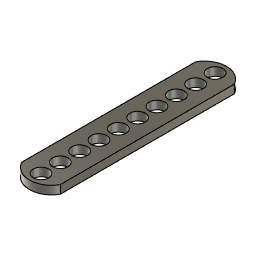
Cut_Link v2 (Autodesk Fusion 360 design; units mm, degrees)
Autodesk Fusion 360 part; units mm, degrees
sketch "Sketch1" plane through (0, 0, 0) normal (0, 0, 1) x (1, 0, 0)
  line L0 (0, 0) -> (0, 45) construction
  line L1 (0, 0) -> (-5, 0)
  line L2 (-5, 0) -> (-5, 45)
  line L3 (-5, 45) -> (0, 45)
  line L4 (5, 0) -> (5, 45)
  line L5 (0, 22.5) -> (9.3523, 22.5) construction
  arc A0 (5, 45) -> (-5, 45) centre (0, 42.289) ccw
  circle A1 centre (0, 45) radius 2
  arc A2 (-5, 0) -> (5, 0) centre (0, 2.711) ccw
  circle A3 centre (0, 0) radius 2
  circle A4 centre (0, 40) radius 2
  circle A5 centre (0, 35) radius 2
  circle A6 centre (0, 30) radius 2
  circle A7 centre (0, 25) radius 2
  circle A8 centre (0, 5) radius 2
  circle A9 centre (0, 10) radius 2
  circle A10 centre (0, 15) radius 2
  circle A11 centre (0, 20) radius 2
  dimension "d1" = 45
  dimension "d2" = 5
  dimension "d3" = 45
  dimension "d4" = 4
  dimension "d7" = 4
  dimension "d8" = 4
  dimension "d9" = 4
  dimension "d10" = 4
  constraint coincident L0.start L1.start
  constraint vertical L0
  constraint horizontal L1
  constraint vertical L2
  constraint horizontal L3
  constraint symmetric L0 L1.end L4.start
  constraint symmetric L0 L2.end L4.end
  constraint midpoint L0 L5.start
  constraint perpendicular L4 L5
  constraint coincident L0.end L3.end
  constraint symmetric L2.end L5 L1.end
  constraint symmetric L4.end L5 L4.start
  constraint symmetric L5 A0 A2
  constraint symmetric L5 A1 A3
  constraint symmetric L5 A4 A8
  constraint symmetric L5 A5 A9
  constraint symmetric L5 A6 A10
  constraint symmetric L5 A7 A11
  measures "d1" distance of L0.start L0.end
  measures "d2" distance of L0.start L1.end
  measures "d3" distance of L0.start L0.end
  measures "d4" diameter of A1
  measures "d7" diameter of A4
  measures "d8" diameter of A5
  measures "d9" diameter of A6
  measures "d10" diameter of A7
extrude "Extrude1" add sketch "Sketch1" along normal blind 2.15 contours L2 L4 A0 A2 | A4 | A5 | A6 | A7 | A8 | A9 | A10 | A11
extrude "Extrude2" cut sketch "Sketch1" along normal up to surface (2.15 mm away) contours A4 | A5 | A6 | A7 | A8 | A9 | A10 | A11
